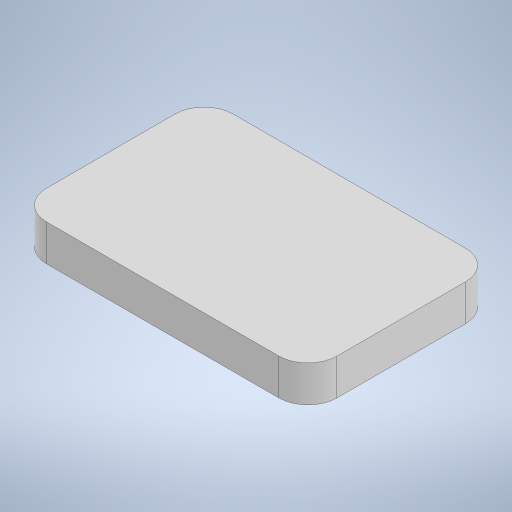
# Autodesk Inventor part: sidemotor
Saved by Autodesk Inventor 2023.2 (Build 272271000, 271)
## iProperties
Created: 2022-12-08
Part Number: sidemotor
Material: Generic
Document SubType Name: Modeling
Designer: kakik
Density: 1 g/cm^3
Appearance: Default
Author: kakik
Autodesk Inventor part; units mm, degrees
ref_plane "YZ Plane" through (0, 0, 0) normal (1, 0, 0) x (0, 1, 0)
ref_plane "XZ Plane" through (0, 0, 0) normal (0, 1, 0) x (-1, 0, 0)
ref_plane "XY Plane" through (0, 0, 0) normal (0, 0, 1) x (1, 0, 0)
sketch "Sketch1" plane through (0, 0, 0) normal (0, 1, 0) x (-1, 0, 0)
  line L0 (8, 6.425) -> (-8, 6.425)
  line L1 (-10, 4.425) -> (-10, -4.425)
  line L2 (-8, -6.425) -> (8, -6.425)
  line L3 (10, -4.425) -> (10, 4.425)
  line L4 (10, 6.425) -> (-10, -6.425) construction
  line L5 (-10, 6.425) -> (10, -6.425) construction
  arc A0 (10, 4.425) -> (8, 6.425) centre (8, 4.425) ccw
  arc A1 (-8, 6.425) -> (-10, 4.425) centre (-8, 4.425) ccw
  arc A2 (-10, -4.425) -> (-8, -6.425) centre (-8, -4.425) ccw
  arc A3 (8, -6.425) -> (10, -4.425) centre (8, -4.425) ccw
  point P0 (0, 0)
  dimension "d0" = 12.85
  dimension "d1" = 20
  dimension "d2" = 2
  constraints: 12 end point, 8 point on circle, 8 point on line, 8 tangent, 4 centre point, 3 equal radius, 2 midpoint, 2 parallel, 1 horizontal, 1 perpendicular
  measures "d0" distance of L5.end L4.start
  measures "d1" distance of L4.end L5.end
  measures "d2" radius of A0
extrude "Extrusion1" add sketch "Sketch1" along normal blind 2.5
body "Solid1"
